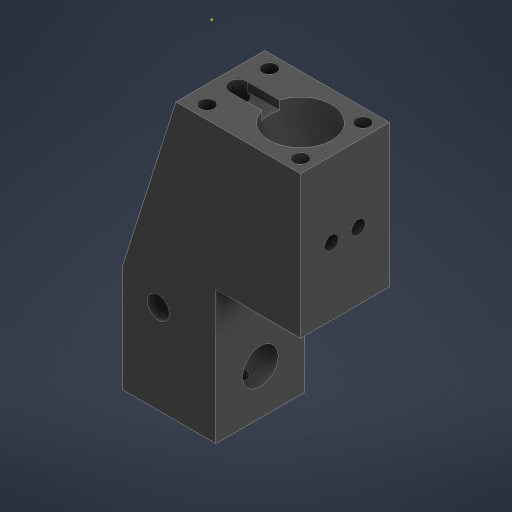
# Autodesk Inventor part: MOTORBLOCK PART 3
Saved by Autodesk Inventor 2023 (Build 270158000, 158)
## iProperties
Created: 2020-07-02
Part Number: MOTORBLOCK PART 3
Material: Steel ASTM A36
Document SubType Name: Modeling
Designer: Smit Ambardekar
Density: 7.85 g/cm^3
Appearance: Generic
Author: Smit Ambardekar
Autodesk Inventor part; units mm, degrees
ref_plane "YZ Plane" through (0, 0, 0) normal (1, 0, 0) x (0, 1, 0)
ref_plane "XZ Plane" through (0, 0, 0) normal (0, 1, 0) x (-1, 0, 0)
sketch "Sketch1" plane through (0, 0, 0) normal (0, 0, 1) x (1, 0, 0)
  line L0 (0, 0) -> (0, 24)
  line L1 (0, 0) -> (21, 0)
  line L2 (21, 0) -> (21, 30)
  line L3 (21, 30) -> (40, 30)
  line L4 (40, 30) -> (40, 62)
  line L5 (40, 62) -> (12, 62)
  line L6 (12, 62) -> (0, 24)
  dimension "d0" = 24
  dimension "d1" = 21
  dimension "d2" = 30
  dimension "d3" = 19
  dimension "d4" = 32
  dimension "d5" = 28
  constraints: 14 end point, 4 perpendicular, 1 horizontal, 1 vertical
  measures "d0" distance of L0.start L0.end
  measures "d1" distance of L0.start L1.end
  measures "d2" distance of L1.end L2.end
  measures "d3" distance of L2.end L3.end
  measures "d4" distance of L3.end L4.end
  measures "d5" distance of L4.end L5.end
extrude "Extrusion1" add sketch "Sketch1" along normal blind 20
sketch "Sketch2" plane through (12, 62, 0) normal (0, 1, 0) x (1, 0, 0)
  line L0 (28, 0) -> (28, -20) projected
  line L1 (28, -10) -> (18, -10)
  line L2 (28, 0) -> (28, -20) projected
  line L3 (28, -20) -> (0, -20) projected
  line L4 (0, -20) -> (0, 0) projected
  line L5 (0, 0) -> (28, 0) projected
  line L6 (28, 0) -> (28, -20) projected
  line L7 (28, -20) -> (0, -20) projected
  line L8 (0, -20) -> (0, 0) projected
  line L9 (0, 0) -> (28, 0) projected
  circle A0 centre (24, -17) radius 1.5
  circle A1 centre (24, -3) radius 1.5
  circle A2 centre (4, -3) radius 1.5
  circle A3 centre (4, -17) radius 1.5
  point P0 (-12, 0)
  point P1 (14, -10)
  dimension "d8" = 10
  dimension "d18" = 3
  dimension "d19" = 3
  dimension "d20" = 3
  constraints: 4 centre point, 2 end point, 1 horizontal, 1 midpoint
  measures "d8" distance of L1.start L1.end
  measures "d18" diameter of A0
  measures "d19" diameter of A1
  measures "d20" diameter of A2
hole "Hole1" at (30, 62, 10) direction (0, -1, 0) diameter 14 end through all
sketch "Sketch3" plane through (12, 62, 0) normal (0, 1, 0) x (1, 0, 0)
  line L0 (28, 0) -> (28, -20) projected
  line L1 (28, -20) -> (25, -20)
  line L2 (28, -20) -> (0, -20) projected
  line L3 (25, -20) -> (25, 0)
  line L4 (28, 0) -> (0, 0) projected
  line L5 (25, 0) -> (4, 0)
  line L6 (4, 0) -> (4, -20)
  line L7 (4, -20) -> (25, -20)
  line L8 (4, -10) -> (4, -17)
  line L9 (4, -17) -> (25, -17)
  line L10 (25, -17) -> (25, -3)
  line L11 (25, -3) -> (4, -3)
  point P0 (-12, 0)
  dimension "d21" = 3
  dimension "d22" = 21
  dimension "d23" = 7
  constraints: 18 end point, 7 point on line, 6 perpendicular, 1 midpoint
  measures "d21" distance of L0.end L1.end
  measures "d22" distance of L3.end L5.end
  measures "d23" distance of L8.start L8.end
hole "Hole2" at (37, 62, 17) at (37, 62, 3) at (16, 62, 3) at (16, 62, 17) direction (0, -1, 0) diameter 3.2 depth 6
sketch "Sketch4" plane through (12, 62, 0) normal (0, 1, 0) x (1, 0, 0)
  point P0 (-12, 0)
sketch "Sketch5" plane through (12, 62, 0) normal (0, 1, 0) x (1, 0, 0)
  circle A0 centre (18, -10) radius 7 projected
  circle A1 centre (4, -10) radius 2
  line L0 (4, -12) -> (11.2918, -12)
  line L1 (4, -8) -> (11.2918, -8)
  point P0 (-12, 0)
  dimension "d32" = 4
  constraints: 4 end point, 4 point on circle, 2 tangent, 1 centre point, 1 horizontal, 1 parallel
  measures "d32" diameter of A1
extrude "Extrusion2" cut sketch "Sketch5" against normal blind 2 contours A0 L0 A1 L1
sketch "Sketch6" plane through (12, 62, 0) normal (0, 1, 0) x (1, 0, 0)
  arc A0 (4, -12) -> (4, -8) centre (4, -10) ccw projected
  circle A1 centre (4, -10) radius 2
  point P0 (-12, 0)
  constraints: 1 centre point, 1 coincident
extrude "Extrusion3" cut sketch "Sketch6" against normal blind 30
sketch "Sketch7" plane through (0, 0, 0) normal (-1, 0, 0) x (0, 0, 1)
  line L0 (0, 0) -> (20, 0) projected
  line L1 (10, 0) -> (10, 10)
  dimension "d37" = 10
  constraints: 2 end point, 1 midpoint, 1 vertical
  measures "d37" distance of L1.start L1.end
hole "Hole3" at (0, 10, 10) direction (1, 0, 0) diameter 8 end through all countersink diameter 10 countersink angle 90
sketch "Sketch8" plane through (0, 0, 20) normal (0, 0, 1) x (1, 0, 0)
  line L0 (0, 24) -> (0, 0) projected
  line L1 (0, 0) -> (0, 20)
  line L2 (0, 20) -> (8, 20)
  dimension "d45" = 20
  dimension "d46" = 8
  constraints: 4 end point, 1 horizontal, 1 point on line
  measures "d45" distance of L0.end L1.end
  measures "d46" distance of L1.end L2.end
hole "Hole4" at (8, 20, 20) direction (0, 0, -1) diameter 5 end through all
ref_plane "Work Plane1" through (12, 32, 0) normal (0, 1, 0) x (1, 0, 0)
sketch "Sketch9" plane through (12, 32, 0) normal (0, 1, 0) x (1, 0, 0)
  arc A0 (4, -12) -> (4, -8) centre (4, -10) ccw projected
  circle A1 centre (4, -10) radius 1.25
  point P0 (-12, 0)
  dimension "d55" = 2.5
  constraints: 1 centre point, 1 coincident
  measures "d55" diameter of A1
hole "Hole5" at (16, 32, 10) direction (0, -1, 0) diameter 2.5 depth 18 tip angle 118
hole "Hole6" at (16, 62, 17) at (37, 62, 17) at (37, 62, 3) at (16, 62, 3) direction (0, -1, 0) diameter 3 depth 9 tip angle 118
hole "Hole7" at (16, 62, 17) at (37, 62, 17) at (37, 62, 3) at (16, 62, 3) direction (0, -1, 0) diameter 3 depth 9 tip angle 118
sketch "Sketch10" plane through (0, 0, 0) normal (0, -1, 0) x (1, 0, 0)
  line L0 (0, 5) -> (0, 15) projected
  line L1 (0, 10) -> (8, 10)
  arc A0 (16, 12) -> (16, 8) centre (16, 10) ccw projected
  line L2 (8, 10) -> (16, 10)
  point P0 (0, 0)
  dimension "d77" = 8
  dimension "d78" = 8
  constraints: 4 end point, 1 collinear, 1 horizontal, 1 midpoint
  measures "d77" distance of L1.start L1.end
  measures "d78" distance of L1.end L2.end
hole "Hole8" at (8, 0, 10) at (16, 0, 10) direction (0, 1, 0) diameter 4 depth 6 tip angle 118
sketch "Sketch11" plane through (40, 30, 0) normal (1, 0, 0) x (0, 0, -1)
  line L0 (-12, 32) -> (-8, 32) projected
  line L1 (-10, 32) -> (-10, 15)
  line L2 (-10, 15) -> (-13, 15)
  line L3 (-13, 15) -> (-7, 15)
  point P0 (0, -30)
  dimension "d86" = 17
  dimension "d87" = 3
  dimension "d88" = 6
  constraints: 6 end point, 1 midpoint, 1 perpendicular, 1 point on line, 1 vertical
  measures "d86" distance of L1.start L1.end
  measures "d87" distance of L1.end L2.end
  measures "d88" distance of L2.end L3.end
hole "Hole9" at (40, 45, 13) at (40, 45, 7) direction (-1, 0, 0) diameter 3.2 depth 3 tip angle 118
body "Solid1"
